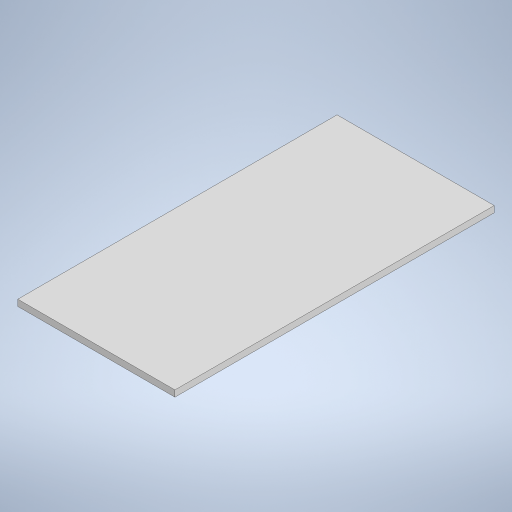
# Autodesk Inventor part: Part2
Saved by Autodesk Inventor 2024 (Build 280153000, 153)
## iProperties
Created: 2024-05-27
Part Number: Part2
Material: Generic
Document SubType Name: Modeling
Designer: samue
Density: 1 g/cm^3
Appearance: Default
Author: samue
Autodesk Inventor part; units mm, degrees
ref_plane "YZ Plane" through (0, 0, 0) normal (1, 0, 0) x (0, 1, 0)
ref_plane "XZ Plane" through (0, 0, 0) normal (0, 1, 0) x (-1, 0, 0)
ref_plane "XY Plane" through (0, 0, 0) normal (0, 0, 1) x (1, 0, 0)
sketch "Sketch1" plane through (0, 0, 0) normal (0, 1, 0) x (-1, 0, 0)
  line L0 (25, 50.8) -> (-25, 50.8)
  line L1 (-25, 50.8) -> (-25, -50.8)
  line L2 (-25, -50.8) -> (25, -50.8)
  line L3 (25, -50.8) -> (25, 50.8)
  line L4 (25, 50.8) -> (-25, -50.8) construction
  line L5 (-25, 50.8) -> (25, -50.8) construction
  point P0 (0, 0)
  dimension "d0" = 101.6
  dimension "d1" = 50
  constraints: 12 end point, 2 midpoint, 2 parallel, 1 horizontal, 1 perpendicular
  measures "d0" distance of L1.end L0.end
  measures "d1" distance of L1.end L2.end
extrude "Extrusion1" add sketch "Sketch1" along normal blind 2
body "Solid1"
